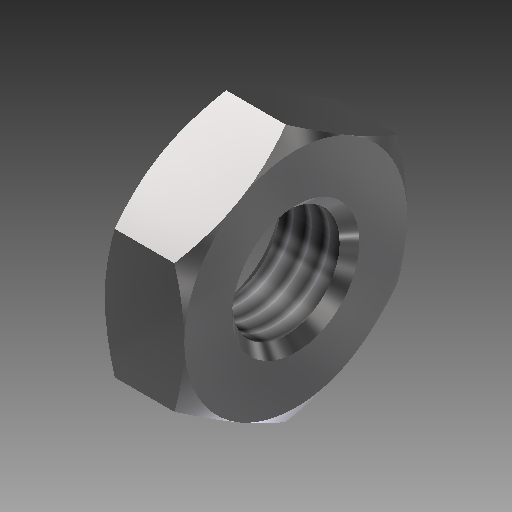
# Autodesk Inventor part: PN1972-015_NUT1/4-28-UNF
Saved by Autodesk Inventor 2017 (Build 210142000, 142)
## iProperties
Category: PARTsolutions
Company: PHD
Created: 2015-12-03
Part Number: PN1972-015_NUT1/4-28-UNF
Catalog Web Link: www.cadenas.de
Description: 1972_Imperial_Nut-Imperial Nut
Vendor: PHD
Document SubType Name: Modeling
Designer: psAdmin
Manufacturer: PHD
Mass: 2.61447 g
Surface Area: 3.68877 cm^2
Volume: 0.326809 cm^3
Density: 8 g/cm^3
Material: Stainless Steel
Appearance: Semi-Polished
PSOL_IDENT_0: {$CADENAS_DATA\23d-libs\phd\fasteners_imp\nuts\1972_nut.prj},201 {VTYP=3D},{NB=PN1972-015_NUT1/4-28-
PSOL_IDENT_1: UNF},{LINA=PN1972-015_NUT1/4-28-UNF},{NN=1972_Imperial_Nut},{DATE=20.11.2015 15:31:40},{GEOMDATE=03.
PSOL_IDENT_2: 12.2013 19:03:23},{VERSION=},{LINEID=20},{LINESUBID=-1},{WBVAR=}  {NB=PN1972-015_NUT1/4-28-UNF},{LIN
PSOL_IDENT_3: A=PN1972-015_NUT1/4-28-UNF},{KT=DUMMY},{IDNR=nut},{DESC=hex jam nut},{DASHNO=015},{PHDPARTNO=1972-01
PSOL_IDENT_4: 5},{THREAD=1/4-28},{THDTYPE=UNF},{THDDIA=0.2500},{HEX=0.4375},{HGHT=0.1560},{CHAMF=30.0},{A=0.000},{
PSOL_IDENT_5: B=0.000},{RAD=0.000}
NN: 1972_Imperial_Nut
NT: Imperial Nut
NB: PN1972-015_NUT1/4-28-UNF
NBSYN: PN$PHDPARTNO._NUT$THREAD.-$THDTYPE.
LINA: PN1972-015_NUT1/4-28-UNF
IDNR: nut
DESC: hex jam nut
DASHNO: 015
PHDPARTNO: 1972-015
THREAD: 1/4-28
THDTYPE: UNF
THDDIA: 0.2500
HEX: 0.4375
HGHT: 0.1560
CHAMF: 30.0
A: 0.000
B: 0.000
RAD: 0.000
SUPPLIER: PHD
ARTICLENO: PN1972-015_NUT1/4-28-UNF
BOMINFO: PN1972-015_NUT1/4-28-UNF
CREATOR: CADENAS GmbH
Title: PN1972-015_NUT1/4-28-UNF
Author: Cadenas PARTsolutions
Comments: Imperial Nut
Autodesk Inventor part; units mm, degrees
sketch "Sketch_1" plane through (0, 0, 0) normal (1, 0, 0) x (0, 1, 0)
  line L0 (-3.2079, 5.5563) -> (-6.4158, 0)
  line L1 (-6.4158, 0) -> (-3.2079, -5.5563)
  line L2 (-3.2079, -5.5563) -> (3.2079, -5.5563)
  line L3 (3.2079, -5.5563) -> (6.4158, 0)
  line L4 (6.4158, 0) -> (3.2079, 5.5563)
  line L5 (3.2079, 5.5563) -> (-3.2079, 5.5563)
  constraints: 12 end point
extrude "Extrusion1" add sketch "Sketch_1" along normal blind 3.9624
sketch "Fine_Thread" plane through (0, 0, 0) normal (0, 0, 1) x (1, 0, 0)
  line L0 (3.9624, 0) -> (0, 0)
  line L1 (0, 0) -> (0, 3.175)
  line L2 (0, 3.175) -> (0.4915, 2.6835)
  line L3 (0.4915, 2.6835) -> (3.4709, 2.6835)
  line L4 (3.4709, 2.6835) -> (3.9624, 3.175)
  line L5 (3.9624, 3.175) -> (3.9624, 0)
  line L6 (3.9624, 0) -> (0, 0)
  constraints: 14 end point
revolve "Revolution1" cut sketch "Fine_Thread" angle 360 about axis through (3.9624, 0, 0) along (1, 0, 0)
thread "Thread1" size "1/4-28 UNF" class "2B" standard "ANSI Unified Screw Threads" full length
sketch "Sketch_3" plane through (0, 0, 0) normal (0, 0, 1) x (1, 0, 0)
  line L0 (25.4, 0) -> (-25.4, 0)
  line L1 (-0.508, 5.5563) -> (0, 5.5563)
  line L2 (0, 5.5563) -> (1.9812, 8.9878)
  line L3 (1.9812, 8.9878) -> (3.9624, 5.5563)
  line L4 (3.9624, 5.5563) -> (4.4704, 5.5563)
  line L5 (4.4704, 5.5563) -> (4.4704, 56.3563)
  line L6 (4.4704, 56.3563) -> (-0.508, 56.3563)
  line L7 (-0.508, 56.3563) -> (-0.508, 5.5563)
  constraints: 16 end point
revolve "Revolution2" cut sketch "Sketch_3" angle 360 about axis through (25.4, 0, 0) along (1, 0, 0)
ref_plane "conn_XY" through (0, 0, 0) normal (1, 0, 0) x (0, 0, -1)
ref_plane "conn_YZ" through (0, 0, 0) normal (0, 0, -1) x (0, 1, 0)
ref_plane "conn_ZX" through (0, 0, 0) normal (0, 1, 0) x (1, 0, 0)
body "Solid1"
